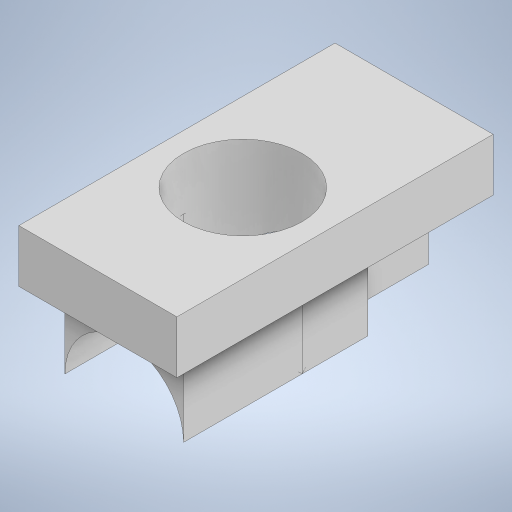
# Autodesk Inventor part: housing_lid_V2
Saved by Autodesk Inventor 2023 (Build 270158000, 158)
## iProperties
Created: 2023-03-23
Part Number: housing_lid_V2
Material: Generic
Document SubType Name: Modeling
Designer: caleb
Density: 1 g/cm^3
Appearance: Default
Author: caleb
Autodesk Inventor part; units mm, degrees
ref_plane "YZ Plane" through (0, 0, 0) normal (1, 0, 0) x (0, 1, 0)
sketch "Sketch1" plane through (0, 0, 0) normal (0, 1, 0) x (-1, 0, 0)
  line L0 (0, 0) -> (60, 0)
  line L1 (60, 0) -> (60, -120)
  line L2 (60, -120) -> (0, -120)
  line L3 (0, -120) -> (0, 0)
  line L4 (30, -120) -> (30, 0)
  circle A0 centre (30, -55) radius 22.5
  line L5 (19.5, -90) -> (19.5, -115)
  line L6 (19.5, -115) -> (40.5, -115)
  line L7 (40.5, -115) -> (40.5, -90)
  line L8 (40.5, -90) -> (19.5, -90)
  line L9 (19.5, -90) -> (40.5, -115) construction
  line L10 (19.5, -115) -> (40.5, -90) construction
  line L11 (19.5, -90) -> (44.5, -90) construction
  line L12 (25, -80) -> (25, -90)
  line L13 (25, -90) -> (35, -90)
  line L14 (35, -90) -> (35, -80)
  line L15 (35, -80) -> (25, -80)
  line L16 (25, -80) -> (35, -90) construction
  line L17 (25, -90) -> (35, -80) construction
  line L18 (25, -80) -> (35, -80) construction
  line L19 (7.5, -10) -> (7.5, -80)
  line L20 (7.5, -80) -> (52.5, -80)
  line L21 (52.5, -80) -> (52.5, -10)
  line L22 (52.5, -10) -> (7.5, -10)
  line L23 (7.5, -10) -> (52.5, -80) construction
  line L24 (7.5, -80) -> (52.5, -10) construction
  line L25 (7.5, -10) -> (77.5, -10) construction
  point P0 (30, -115)
  point P1 (30, -90)
  point P2 (30, -90)
  point P3 (30, -80)
  point P4 (30, -77.5)
  point P5 (30, -25)
  point P6 (30, -102.5)
  point P7 (30, -10)
  point P8 (30, -85)
  point P9 (30, -10)
  point P10 (30, -45)
  point P11 (25, -90)
  point P12 (35, -90)
  point P13 (35, -80)
  point P14 (25, -80)
  dimension "d0" = 60
  dimension "d1" = 120
  dimension "d2" = 45
  dimension "d3" = 5
  dimension "d4" = 25
  dimension "d5" = 0
  dimension "d6" = 12.5
  dimension "d7" = 10
  dimension "d8" = 2.5
  dimension "d9" = 22.5
  dimension "d10" = -70
  dimension "d11" = 25
  dimension "d12" = 90
  dimension "d13" = 21
  dimension "d14" = 5
  dimension "d15" = 10
  dimension "d16" = 90
  dimension "d17" = 10
  dimension "d19" = -70
  dimension "d20" = 90
  dimension "d21" = -35
  dimension "d22" = 45
  constraints: 52 end point, 11 parallel, 8 midpoint, 7 perpendicular, 5 point on line, 4 horizontal, 2 coincident, 1 centre point
  measures "d0" distance of L1.end L2.end
  measures "d1" distance of L0.end L1.end
  measures "d2" diameter of A0
  measures "d3" distance from line of L2 point (30, -115)
  measures "d4" distance of point (30, -90) point (30, -115)
  measures "d5" distance of point (30, -90) point (30, -90)
  measures "d6" distance of point (30, -115) point (30, -102.5)
  measures "d7" distance of point (30, -80) point (30, -90)
  measures "d8" distance of point (30, -77.5) point (30, -80)
  measures "d9" distance of point (30, -55) point (30, -77.5)
  measures "d10" distance of point (30, -10) point (30, -80)
  measures "d11" distance of L5.start L5.end
  measures "d12" angle of L5 L11
  measures "d13" distance of L6.end L5.end
  measures "d14" distance of point (30, -85) point (30, -90)
  measures "d15" distance of L12.start L12.end
  measures "d16" angle of L12 L18
  measures "d17" distance of L13.end L12.end
  measures "d19" distance of L19.start L19.end
  measures "d20" angle of L19 L25
  measures "d21" distance of point (30, -80) point (30, -45)
  measures "d22" distance between parallel lines of L19 L21
extrude "Extrusion1" add sketch "Sketch1" along normal blind 20
ref_plane "Work Plane1" through (0, 20, -120) normal (0, 0, -1) x (-1, 0, 0)
sketch "Sketch2" plane through (0, 20, -120) normal (0, 0, -1) x (-1, 0, 0)
  line L0 (0, -20) -> (60, -20) projected
  line L1 (60, -20) -> (60, 0) projected
  line L2 (0, 0) -> (60, 0) projected
  line L3 (0, -20) -> (0, 0) projected
  line L4 (60, -20) -> (0, -20) projected
  line L5 (0, -20) -> (60, -20)
  line L6 (60, -20) -> (60, -80)
  line L7 (60, -80) -> (0, -80)
  line L8 (0, -80) -> (0, -20)
  point P0 (30, -50)
  dimension "d25" = 60
  dimension "d26" = 60
  dimension "d27" = 30
  dimension "d28" = 30
  constraints: 8 end point, 2 parallel, 1 horizontal, 1 perpendicular
  measures "d25" distance of L6.end L7.end
  measures "d26" distance of L5.end L6.end
  measures "d27" distance from line of L7 point (30, -50)
  measures "d28" distance from line of L6 point (30, -50)
ref_plane "Work Plane2" through (-30, -30, -120) normal (0, 1, 0) x (1, 0, 0)
extrude "Extrusion2" add sketch "Sketch1" against normal up to surface (30 mm away) contours L22 L21 A0 L4 | L4 A0 L19 L22 | A0 L4 | L4 A0 | L6 L5 L8 L4 | L4 L8 L7 L6 | A0 L21 L20 L15 L4 | L4 L15 L20 L19 A0 | L8 L12 L15 L4 | L4 L15 L14 L8
extrude "Extrusion3" cut sketch "Sketch1" along normal through all both and the other way through all contours A0 L4 | L4 A0
ref_plane "Work Plane6" through (-7.5, -30, -10) normal (0, 0, -1) x (-1, 0, 0)
ref_plane "Work Plane5" through (-7.5, -30, -80) normal (0, 0, -1) x (-1, 0, 0)
sketch "Sketch3" plane through (-40.5, -30, -115) normal (0, 0, -1) x (-1, 0, 0)
  line L0 (0, 30) -> (0, 0) projected
  circle A0 centre (-10.5, 0) radius 10.5
  point P0 (-40.5, 30)
  constraints: 1 coincident, 1 horizontal alignment, 2 other
sketch "Sketch4" plane through (-19.5, -30, -90) normal (0, 0, -1) x (-1, 0, 0)
  line L0 (5.5, 30) -> (5.5, 0) projected
  line L1 (15.5, 30) -> (15.5, 0) projected
  circle A0 centre (10.5, 0) radius 5
  point P0 (-19.5, 30)
  constraints: 1 coincident, 1 horizontal alignment, 2 other
sketch "Sketch5" plane through (-7.5, -30, -80) normal (0, 0, -1) x (-1, 0, 0)
  line L0 (0, 50) -> (45, 50) projected
  circle A0 centre (22.5, 0) radius 22.5
  point P0 (-7.5, 30)
  constraints: 1 centre point, 1 coincident
extrude "Extrusion4" cut sketch "Sketch3" against normal up to surface (25 mm away)
extrude "Extrusion5" cut sketch "Sketch5" against normal up to surface (70 mm away)
extrude "Extrusion6" cut sketch "Sketch4" against normal up to surface (10 mm away)
ref_plane "Work Plane3" through (-40.5, -30, -115) normal (0, 0, -1) x (-1, 0, 0)
ref_plane "Work Plane4" through (-19.5, -30, -90) normal (0, 0, -1) x (-1, 0, 0)
equation "\"d4\" = d11"
equation "\"d6\" = 0.5 * d4"
equation "\"d7\" = d15"
equation "\"d9\" = 0.5 * d2"
equation "\"d14\" = 0.5 * d7"
equation "\"d19\" = d10"
equation "\"d21\" = 0.5 * d10"
equation "\"d22\" = d2"
equation "\"d25\" = d0"
equation "\"d26\" = d25"
equation "\"d27\" = 0.5 * d26"
equation "\"d28\" = 0.5 * d25"
body "Solid1"
